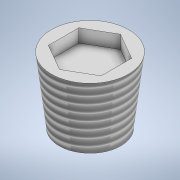
# Autodesk Inventor part: Пробка
Saved by Autodesk Inventor 2021 (Build 250183000, 183)
## iProperties
Created: 2021-04-19
Part Number: Пробка
Material: Типовые
Document SubType Name: Modeling
Designer: Данил
Density: 1 g/cm^3
Appearance: По умолчанию
Author: Данил
Autodesk Inventor part; units mm, degrees
ref_plane "YZ Plane" through (0, 0, 0) normal (1, 0, 0) x (0, 1, 0)
ref_plane "XZ Plane" through (0, 0, 0) normal (0, 1, 0) x (-1, 0, 0)
ref_plane "XY Plane" through (0, 0, 0) normal (0, 0, 1) x (1, 0, 0)
sketch "Эскиз1" plane through (0, 0, 0) normal (0, 0, 1) x (1, 0, 0)
  line L0 (0, 7.5) -> (0, -7.5)
  line L1 (0, 7.5) -> (8.75, 7.5)
  line L2 (8.75, 7.5) -> (7, -7.5)
  line L3 (7, -7.5) -> (0, -7.5)
  point P0 (0, 0)
  point P1 (0, 0)
  dimension "d0" = 15
  dimension "d1" = 17.5
  dimension "d2" = 14
  constraints: 8 end point, 1 coincident, 1 horizontal, 1 midpoint, 1 parallel, 1 vertical
  measures "d0" distance of L0.start L0.end
  measures "d1" diameter of L1.end L0
  measures "d2" diameter of L2.end L0
revolve "Вращение1" add sketch "Эскиз1" angle 360 about axis through (0, 7.5, 0) along (0, -1, 0)
sketch "Эскиз2" plane through (0, 7.5, 0) normal (0, 1, 0) x (1, 0, 0)
  line L0 (0, 6.9282) -> (6, 3.4641)
  line L1 (6, 3.4641) -> (6, -3.4641)
  line L2 (6, -3.4641) -> (0, -6.9282)
  line L3 (0, -6.9282) -> (-6, -3.4641)
  line L4 (-6, -3.4641) -> (-6, 3.4641)
  line L5 (-6, 3.4641) -> (0, 6.9282)
  point P0 (0, 0)
  point P1 (0, 0)
  dimension "d4" = 12
  constraints: 12 end point, 1 coincident, 1 vertical, 13 other
  measures "d4" distance between parallel lines of L1 L4
extrude "Выдавливание1" cut sketch "Эскиз2" against normal blind 3
thread "Резьба1" size "R 1/2" standard "ISO Taper" length 18.2
